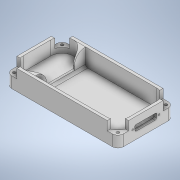
# Autodesk Inventor part: Podstawa
Saved by Autodesk Inventor 2020.3 (Build 243373000, 373)
## iProperties
Created: 2021-03-04
Part Number: Podstawa
Material: Generic
Document SubType Name: Modeling
Designer: patry
Density: 1 g/cm^3
Appearance: Default
Author: patry
Autodesk Inventor part; units mm, degrees
ref_plane "YZ Plane" through (0, 0, 0) normal (1, 0, 0) x (0, 1, 0)
ref_plane "XZ Plane" through (0, 0, 0) normal (0, 1, 0) x (-1, 0, 0)
ref_plane "XY Plane" through (0, 0, 0) normal (0, 0, 1) x (1, 0, 0)
sketch "Sketch2" plane through (0, 0, 0) normal (0, 1, 0) x (-1, 0, 0)
  line L0 (0, 0) -> (-200, 0)
  line L1 (-200, 0) -> (-200, -100)
  line L2 (-200, -100) -> (0, -100)
  line L3 (0, -100) -> (0, 0)
  dimension "d0" = 200
  dimension "d1" = 100
  constraints: 8 end point, 2 parallel, 1 horizontal, 1 perpendicular
  measures "d0" distance of L2.end L1.end
  measures "d1" distance of L1.end L0.end
extrude "Extrusion1" add sketch "Sketch2" along normal blind 11
sketch "Sketch3" plane through (0, 11, 0) normal (0, 1, 0) x (1, 0, 0)
  line L0 (0, 100) -> (0, 0) projected
  line L1 (0, 0) -> (200, 0) projected
  line L2 (0, 100) -> (200, 100)
  line L3 (200, 100) -> (200, 0)
  line L4 (200, 0) -> (0, 0)
  line L5 (0, 0) -> (0, 100)
  line L6 (0, 100) -> (5, 100)
  line L7 (5, 100) -> (5, 95)
  line L8 (5, 95) -> (0, 95)
  line L9 (0, 95) -> (0, 100)
  line L10 (200, 0) -> (195, 0)
  line L11 (195, 0) -> (195, 5)
  line L12 (195, 5) -> (200, 5)
  line L13 (200, 5) -> (200, 0)
  line L14 (5, 95) -> (195, 95)
  line L15 (195, 95) -> (195, 5)
  line L16 (195, 5) -> (5, 5)
  line L17 (5, 5) -> (5, 95)
  dimension "d4" = 5
  dimension "d5" = 5
  dimension "d6" = 5
  dimension "d7" = 5
  constraints: 32 end point, 8 parallel, 4 horizontal, 4 perpendicular
  measures "d4" distance of L7.end L8.end
  measures "d5" distance of L6.end L7.end
  measures "d6" distance of L11.end L12.end
  measures "d7" distance of L10.end L11.end
extrude "Extrusion2" add sketch "Sketch3" along normal blind 25 contours L2 L7 L8 L0 | L8 L17 L16 L11 L1 L0 | L2 L3 L12 L15 L14 L7 | L11 L12 L3 L1
fillet "Fillet1" radius 10 4 edges at (0, 18, -100) (0, 18, 0) (200, 18, 0) (200, 18, -100)
fillet "Fillet2" radius 20 4 edges at (5, 23.5, -95) (5, 23.5, -5) (195, 23.5, -5) (195, 23.5, -95)
sketch "Sketch4" plane through (0, 36, 0) normal (0, 1, 0) x (1, 0, 0)
  line L0 (0, 0) -> (200, 0)
  line L1 (200, 0) -> (200, 100)
  line L2 (200, 100) -> (0, 100)
  line L3 (0, 100) -> (0, 0)
  line L4 (0, 0) -> (7, 0)
  line L5 (7, 0) -> (7, 7)
  line L6 (7, 7) -> (0, 7)
  line L7 (0, 7) -> (0, 0)
  line L8 (200, 100) -> (193, 100)
  line L9 (193, 100) -> (193, 93)
  line L10 (193, 93) -> (200, 93)
  line L11 (200, 93) -> (200, 100)
  line L12 (7, 7) -> (193, 7)
  line L13 (193, 7) -> (193, 93)
  line L14 (193, 93) -> (7, 93)
  line L15 (7, 93) -> (7, 7)
  dimension "d12" = 200
  dimension "d13" = 100
  dimension "d14" = 7
  dimension "d15" = 7
  dimension "d16" = 7
  dimension "d17" = 7
  constraints: 32 end point, 8 parallel, 4 horizontal, 4 perpendicular
  measures "d12" distance of L2.end L1.end
  measures "d13" distance of L1.end L0.end
  measures "d14" distance of L6.end L5.end
  measures "d15" distance of L5.end L4.end
  measures "d16" distance of L10.end L9.end
  measures "d17" distance of L9.end L8.end
hole "Hole1" at (7, 36, -7) at (7, 36, -93) at (193, 36, -93) at (193, 36, -7) direction (0, -1, 0) diameter 5 end through all
sketch "Sketch6" plane through (200, 0, -10) normal (1, 0, 0) x (0, 0, -1)
  line L0 (0, 36) -> (0, 0) projected
  line L1 (80, 0) -> (0, 0) projected
  line L2 (0, 36) -> (80, 36)
  line L3 (80, 36) -> (80, 0)
  line L4 (80, 0) -> (0, 0)
  line L5 (0, 0) -> (0, 36)
  line L6 (0, 36) -> (13.5, 36)
  line L7 (13.5, 36) -> (13.5, 24.25)
  line L8 (13.5, 24.25) -> (0, 24.25)
  line L9 (0, 24.25) -> (0, 36)
  line L10 (80, 0) -> (66.5, 0)
  line L11 (66.5, 0) -> (66.5, 11.75)
  line L12 (66.5, 11.75) -> (80, 11.75)
  line L13 (80, 11.75) -> (80, 0)
  line L14 (13.5, 24.25) -> (66.5, 24.25)
  line L15 (66.5, 24.25) -> (66.5, 11.75)
  line L16 (66.5, 11.75) -> (13.5, 11.75)
  line L17 (13.5, 11.75) -> (13.5, 24.25)
  line L18 (13.5, 24.25) -> (16.5, 24.25)
  line L19 (16.5, 24.25) -> (16.5, 11.75)
  line L20 (16.5, 11.75) -> (13.5, 11.75)
  line L21 (13.5, 11.75) -> (13.5, 24.25)
  line L22 (66.5, 24.25) -> (63.5, 24.25)
  line L23 (63.5, 24.25) -> (63.5, 11.75)
  line L24 (63.5, 11.75) -> (66.5, 11.75)
  line L25 (66.5, 11.75) -> (66.5, 24.25)
  line L26 (13.5, 24.25) -> (16.5, 24.25)
  line L27 (16.5, 24.25) -> (16.5, 18)
  line L28 (16.5, 18) -> (13.5, 18)
  line L29 (13.5, 18) -> (13.5, 24.25)
  line L30 (66.5, 24.25) -> (63.5, 24.25)
  line L31 (63.5, 24.25) -> (63.5, 18)
  line L32 (63.5, 18) -> (66.5, 18)
  line L33 (66.5, 18) -> (66.5, 24.25)
  circle A0 centre (16.5, 18) radius 1.5
  circle A1 centre (63.5, 18) radius 1.5
  line L34 (13.5, 24.25) -> (19.5, 24.25)
  line L35 (19.5, 24.25) -> (19.5, 23.25)
  line L36 (19.5, 23.25) -> (13.5, 23.25)
  line L37 (13.5, 23.25) -> (13.5, 24.25)
  line L38 (66.5, 11.75) -> (60.5, 11.75)
  line L39 (60.5, 11.75) -> (60.5, 12.75)
  line L40 (60.5, 12.75) -> (66.5, 12.75)
  line L41 (66.5, 12.75) -> (66.5, 11.75)
  line L42 (60.5, 12.75) -> (19.5, 12.75)
  line L43 (19.5, 12.75) -> (19.5, 23.25)
  line L44 (19.5, 23.25) -> (60.5, 23.25)
  line L45 (60.5, 23.25) -> (60.5, 12.75)
  line L46 (19.5, 12.75) -> (21, 12.75)
  line L47 (21, 12.75) -> (21, 14.25)
  line L48 (21, 14.25) -> (19.5, 14.25)
  line L49 (19.5, 14.25) -> (19.5, 12.75)
  line L50 (60.5, 12.75) -> (59, 12.75)
  line L51 (59, 12.75) -> (59, 14.25)
  line L52 (59, 14.25) -> (60.5, 14.25)
  line L53 (60.5, 14.25) -> (60.5, 12.75)
  line L54 (19.5, 23.25) -> (21, 12.75)
  line L55 (59, 12.75) -> (60.5, 23.25)
  line L56 (16.5, 18) -> (16.5, 20.35)
  line L57 (16.5, 18) -> (17.675, 20.0352)
  line L58 (16.5, 18) -> (18.85, 18) construction
  line L59 (18.85, 19.3568) -> (18.85, 16.6432)
  line L60 (18.85, 16.6432) -> (16.5, 15.2865)
  line L61 (16.5, 15.2865) -> (14.15, 16.6432)
  line L62 (14.15, 16.6432) -> (14.15, 19.3568)
  line L63 (14.15, 19.3568) -> (16.5, 20.7135)
  line L64 (16.5, 20.7135) -> (18.85, 19.3568)
  line L65 (65.85, 19.3568) -> (65.85, 16.6432)
  line L66 (65.85, 16.6432) -> (63.5, 15.2865)
  line L67 (63.5, 15.2865) -> (61.15, 16.6432)
  line L68 (61.15, 16.6432) -> (61.15, 19.3568)
  line L69 (61.15, 19.3568) -> (63.5, 20.7135)
  line L70 (63.5, 20.7135) -> (65.85, 19.3568)
  line L71 (14.15, 19.3568) -> (14.15, 16.6432)
  line L72 (16.5, 15.2865) -> (14.15, 16.6432)
  line L73 (19.5, 12.75) -> (20.5, 12.75)
  line L74 (20.5, 12.75) -> (20.5, 13.75)
  line L75 (20.5, 13.75) -> (19.5, 13.75)
  line L76 (19.5, 13.75) -> (19.5, 12.75)
  line L77 (19.5, 13.75) -> (60.5, 13.75)
  line L78 (21, 12.75) -> (21.5, 12.75)
  line L79 (19.5, 23.25) -> (20, 23.25)
  line L80 (20, 23.25) -> (21.5, 12.75)
  line L81 (60.5, 23.25) -> (60, 23.25)
  line L82 (59, 12.75) -> (58.5, 12.75)
  line L83 (58.5, 12.75) -> (60, 23.25)
  point P0 (-10, 0)
  point P1 (59, 12.75)
  point P2 (14.15, 18)
  point P3 (20.8571, 13.75)
  point P4 (59.1429, 13.75)
  point P5 (58.6429, 13.75)
  point P6 (21.3571, 13.75)
  dimension "d123" = 186
  dimension "d124" = 86
  dimension "d31" = 36
  dimension "d32" = 80
  dimension "d33" = 13.5
  dimension "d34" = 11.75
  dimension "d35" = 13.5
  dimension "d36" = 11.75
  dimension "d37" = 3
  dimension "d38" = 3
  dimension "d39" = 3
  dimension "d40" = 6.25
  dimension "d41" = 3
  dimension "d42" = 6.25
  dimension "d43" = 3
  dimension "d44" = 3
  dimension "d45" = 6
  dimension "d46" = 1
  dimension "d47" = 6
  dimension "d48" = 1
  dimension "d49" = 1.5
  dimension "d50" = 1.5
  dimension "d51" = 1.5
  dimension "d52" = 1.5
  dimension "d141" = 2.35
  dimension "d142" = 2.35
  dimension "d143" = 60
  dimension "d144" = 1
  dimension "d145" = 1
  dimension "d148" = 0.5
  dimension "d149" = 0.5
  dimension "d150" = 0.5
  dimension "d151" = 0.5
  constraints: 164 end point, 28 parallel, 15 horizontal, 15 perpendicular, 8 point on line, 3 coincident, 2 centre point, 1 equal length, 1 midpoint, 13 other
  measures "d31" distance of L0.start L0.end
  measures "d32" distance of L0.start L2.end
  measures "d33" distance of L7.end L8.end
  measures "d34" distance of L6.end L7.end
  measures "d35" distance of L11.end L12.end
  measures "d36" distance of L10.end L11.end
  measures "d37" distance of L19.end L20.end
  measures "d38" distance of L24.end L23.end
  measures "d39" distance of L27.end L28.end
  measures "d40" distance of L26.end L27.end
  measures "d41" distance of L32.end L31.end
  measures "d42" distance of L31.end L30.end
  measures "d43" diameter of A0
  measures "d44" diameter of A1
  measures "d45" distance of L35.end L36.end
  measures "d46" distance of L34.end L35.end
  measures "d47" distance of L39.end L40.end
  measures "d48" distance of L38.end L39.end
  measures "d49" distance of L48.end L47.end
  measures "d50" distance of L47.end L46.end
  measures "d51" distance of L51.end L52.end
  measures "d52" distance of L50.end L51.end
  measures "d141" distance of L56.start L56.end
  measures "d142" distance of L56.start L57.end
  measures "d143" angle of L58 L57
  measures "d144" distance of L75.end L74.end
  measures "d145" distance of L74.end L73.end
  measures "d148" distance of L46.end L78.end
  measures "d149" distance of L35.end L79.end
  measures "d150" distance of L44.end L81.end
  measures "d151" distance of L50.end L82.end
sketch "Sketch7" plane through (0, 11, 0) normal (0, 1, 0) x (1, 0, 0)
  arc A0 (25, 95) -> (5, 75) centre (25, 75) ccw projected
  line L0 (195, 25) -> (195, 75) projected
  line L1 (5, 75) -> (195, 75)
  line L2 (195, 75) -> (195, 25)
  line L3 (195, 25) -> (5, 25)
  line L4 (5, 25) -> (5, 75)
  arc A1 (175, 5) -> (195, 25) centre (175, 25) ccw projected
  line L5 (195, 25) -> (156.55, 25)
  line L6 (156.55, 25) -> (156.55, 50)
  line L7 (156.55, 50) -> (195, 50)
  line L8 (195, 50) -> (195, 25)
  line L9 (156.55, 50) -> (149.05, 50)
  line L10 (156.55, 50) -> (152.8, 50)
  line L11 (152.8, 50) -> (152.8, 51)
  line L12 (152.8, 51) -> (156.55, 51)
  line L13 (156.55, 51) -> (156.55, 50)
  line L14 (152.8, 50) -> (21.8, 50)
  line L15 (152.8, 50) -> (283.8, 50) construction
  circle A2 centre (21.8, 50) radius 6
  line L16 (21.8, 50) -> (5.7, 50)
  line L17 (5, 32.7) -> (5, 67.3)
  circle A3 centre (25, 75) radius 20
  arc A4 (5, 25) -> (25, 5) centre (25, 25) ccw projected
  circle A5 centre (25, 25) radius 20
  line L18 (45, 108.4163) -> (45, -35.3074)
  line L19 (25, 95) -> (175, 95) projected
  line L20 (25, 95) -> (45, 95)
  line L21 (175, 5) -> (25, 5) projected
  line L22 (25, 5) -> (45, 5)
  line L23 (45, 95) -> (47, 95)
  line L24 (47, 95) -> (47, 93)
  line L25 (47, 93) -> (45, 93)
  line L26 (45, 93) -> (45, 95)
  line L27 (47, 95) -> (45, 95)
  line L28 (45, 95) -> (45, 5)
  line L29 (45, 5) -> (47, 5)
  line L30 (47, 5) -> (47, 95)
  point P0 (0, 0)
  point P1 (47, 25)
  point P2 (45, 25)
  point P3 (45, 75)
  point P4 (47, 75)
  point P5 (25, 5)
  point P6 (45, 25)
  point P7 (45, 75)
  dimension "d56" = 50
  dimension "d57" = 38.45
  dimension "d58" = 25
  dimension "d59" = 7.5
  dimension "d60" = 3.75
  dimension "d61" = 1
  dimension "d63" = 180
  dimension "d64" = 12
  dimension "d115" = 2
  dimension "d116" = 2
  constraints: 56 end point, 10 parallel, 9 horizontal, 5 perpendicular, 4 point on line, 3 centre point, 3 coincident, 1 collinear, 1 concentric, 1 tangent, 1 vertical
  measures "d56" distance of L3.end L1.start
  measures "d57" distance of L6.end L7.end
  measures "d58" distance of L5.end L6.end
  measures "d59" distance of L6.end L9.end
  measures "d60" distance of L11.end L12.end
  measures "d61" distance of L10.end L11.end
  measures "d63" angle of L14 L15
  measures "d64" diameter of A2
  measures "d115" distance of L24.end L25.end
  measures "d116" distance of L23.end L24.end
extrude "Extrusion7" add sketch "Sketch7" along normal blind 25 contours L19 L18 A3 | L18 L25 L30 L1 | L19 L24 L25 L18 | L18 L21 A5 | L3 L30 L21 L18
fillet "Fillet6" radius 20 2 edges at (46, 36, -25) (46, 36, -75)
sketch "Sketch12" plane through (0, 0, 0) normal (0, -1, 0) x (1, 0, 0)
  circle A0 centre (193, -93) radius 2.5 projected
  line L0 (193, -93) -> (193, -97)
  circle A1 centre (7, -7) radius 2.5 projected
  line L1 (193, -93) -> (7, -93)
  line L2 (7, -93) -> (7, -7)
  line L3 (7, -7) -> (193, -7)
  line L4 (193, -7) -> (193, -93)
  line L5 (193, -97) -> (7, -97)
  line L6 (7, -97) -> (7, -11)
  line L7 (7, -11) -> (193, -11)
  line L8 (193, -11) -> (193, -97)
  line L9 (190.6906, -97) -> (188.3812, -93)
  line L10 (188.3812, -93) -> (190.6906, -89)
  line L11 (190.6906, -89) -> (195.3094, -89)
  line L12 (195.3094, -89) -> (197.6188, -93)
  line L13 (197.6188, -93) -> (195.3094, -97)
  line L14 (195.3094, -97) -> (190.6906, -97)
  line L15 (190.6906, -11) -> (188.3812, -7)
  line L16 (188.3812, -7) -> (190.6906, -3)
  line L17 (190.6906, -3) -> (195.3094, -3)
  line L18 (195.3094, -3) -> (197.6188, -7)
  line L19 (197.6188, -7) -> (195.3094, -11)
  line L20 (195.3094, -11) -> (190.6906, -11)
  line L21 (4.6906, -11) -> (2.3812, -7)
  line L22 (2.3812, -7) -> (4.6906, -3)
  line L23 (4.6906, -3) -> (9.3094, -3)
  line L24 (9.3094, -3) -> (11.6188, -7)
  line L25 (11.6188, -7) -> (9.3094, -11)
  line L26 (9.3094, -11) -> (4.6906, -11)
  line L27 (4.6906, -97) -> (2.3812, -93)
  line L28 (2.3812, -93) -> (4.6906, -89)
  line L29 (4.6906, -89) -> (9.3094, -89)
  line L30 (9.3094, -89) -> (11.6188, -93)
  line L31 (11.6188, -93) -> (9.3094, -97)
  line L32 (9.3094, -97) -> (4.6906, -97)
  point P0 (0, 0)
  dimension "d122" = 4
  dimension "d123" = 186
  dimension "d124" = 86
  dimension "d125" = 186
  dimension "d126" = 86
  constraints: 66 end point, 4 coincident, 4 midpoint, 4 parallel, 2 horizontal, 2 perpendicular, 1 vertical, 52 other
  measures "d122" distance of L0.start L0.end
  measures "d123" distance of L0.start L1.end
  measures "d124" distance of L1.end L2.end
  measures "d125" distance of L6.end L7.end
  measures "d126" distance of L5.end L6.end
sketch "Sketch13" plane through (0, 36, 0) normal (0, 1, 0) x (1, 0, 0)
  arc A0 (5, 25) -> (25, 5) centre (25, 25) ccw projected
  circle A1 centre (25, 25) radius 20
  arc A2 (0, 10) -> (10, 0) centre (10, 10) ccw projected
  circle A3 centre (10, 10) radius 10
  line L0 (5.8856, 19.1144) -> (0, 19.1144)
  line L1 (0, 90) -> (0, 10) projected
  line L2 (19.1144, 5.8856) -> (19.1144, 0)
  line L3 (10, 0) -> (190, 0) projected
  line L4 (0, 19.1144) -> (19.1144, 19.1144)
  line L5 (19.1144, 19.1144) -> (19.1144, 0)
  line L6 (19.1144, 0) -> (0, 0)
  line L7 (0, 0) -> (0, 19.1144)
  arc A4 (45, 75) -> (5, 75) centre (25, 75) ccw projected
  circle A5 centre (25, 75) radius 20
  line L8 (25, 75) -> (25, 25)
  line L9 (25, 75) -> (35, 75)
  line L10 (35, 75) -> (35, 50)
  line L11 (35, 50) -> (25, 50)
  line L12 (25, 50) -> (25, 75)
  circle A6 centre (25, 75) radius 20
  circle A7 centre (10, 90) radius 10
  line L13 (0, 80.8856) -> (19.1144, 80.8856)
  line L14 (19.1144, 80.8856) -> (19.1144, 100)
  line L15 (19.1144, 100) -> (0, 100)
  line L16 (0, 100) -> (0, 80.8856)
  line L17 (0, 100) -> (200, 100)
  line L18 (200, 100) -> (200, 0)
  line L19 (200, 0) -> (0, 0)
  line L20 (0, 0) -> (0, 100)
  line L21 (0, 100) -> (100, 100)
  line L22 (100, 100) -> (100, 0)
  line L23 (100, 0) -> (0, 0)
  line L24 (0, 0) -> (0, 100)
  arc A8 (175, 5) -> (195, 25) centre (175, 25) ccw
  circle A9 centre (175, 25) radius 20
  arc A10 (190, 0) -> (200, 10) centre (190, 10) ccw
  circle A11 centre (190, 10) radius 10
  line L25 (194.1144, 19.1144) -> (200, 19.1144)
  line L26 (200, 90) -> (200, 10)
  line L27 (180.8856, 5.8856) -> (180.8856, 0)
  line L28 (200, 19.1144) -> (180.8856, 19.1144)
  line L29 (180.8856, 19.1144) -> (180.8856, 0)
  line L30 (180.8856, 0) -> (200, 0)
  line L31 (200, 0) -> (200, 19.1144)
  arc A12 (195, 75) -> (155, 75) centre (175, 75) ccw
  circle A13 centre (175, 75) radius 20
  line L32 (175, 75) -> (175, 25)
  line L33 (175, 75) -> (165, 75)
  line L34 (165, 75) -> (165, 50)
  line L35 (165, 50) -> (175, 50)
  line L36 (175, 50) -> (175, 75)
  circle A14 centre (175, 75) radius 20
  line L37 (180.8856, 80.8856) -> (180.8856, 100)
  line L38 (200, 80.8856) -> (180.8856, 80.8856)
  line L39 (200, 100) -> (200, 80.8856)
  line L40 (180.8856, 100) -> (200, 100)
  circle A15 centre (190, 90) radius 10
  line L41 (200, 0) -> (200, 100)
  line L42 (200, 0) -> (200, 100)
  point P0 (19.1144, 5.8856)
  point P1 (5.8856, 19.1144)
  point P2 (10, 100)
  point P3 (5.8856, 80.8856)
  point P4 (19.1144, 94.1144)
  point P5 (180.8856, 5.8856)
  point P6 (180.8856, 94.1144)
  point P7 (194.1144, 80.8856)
  point P8 (190, 100)
  dimension "d131" = 10
  dimension "d132" = 25
  dimension "d133" = 200
  dimension "d134" = 100
  dimension "d135" = 100
  dimension "d136" = 100
  constraints: 82 end point, 35 symmetric about line, 14 point on circle, 13 centre point, 8 parallel, 6 coincident, 5 horizontal, 5 perpendicular, 3 point on line, 1 vertical, 10 other
  measures "d131" distance of L10.end L11.end
  measures "d132" distance of L9.end L10.end
  measures "d133" distance of L18.end L19.end
  measures "d134" distance of L17.end L18.end
  measures "d135" distance of L22.end L23.end
  measures "d136" distance of L21.end L22.end
extrude "Extrusion9" cut sketch "Sketch13" against normal blind 16 contours A0 A3 A2 | A3 L1 L0 | L2 L3 A3 | L1 A7 L13 | A7 A4 | L27 A11 L3 | L15 L14 A7 | A11 A8 A10 | L17 A15 L37 | A11 L25 L18 | A15 A12 | L18 L38 A15
sketch "Sketch15" plane through (0, 11, 0) normal (0, 1, 0) x (1, 0, 0)
  line L0 (47, 95) -> (175, 95) projected
  line L1 (195, 25) -> (195, 75) projected
  line L2 (47, 95) -> (195, 95)
  line L3 (195, 95) -> (195, 52.6168)
  line L4 (195, 52.6168) -> (47, 52.6168)
  line L5 (47, 52.6168) -> (47, 95)
  line L6 (47, 5) -> (175, 5) projected
  line L7 (47, 5) -> (195, 5)
  line L8 (195, 5) -> (195, 52.6168)
  line L9 (195, 52.6168) -> (47, 52.6168)
  line L10 (47, 52.6168) -> (47, 5)
  arc A0 (175, 5) -> (195, 25) centre (175, 25) ccw projected
  circle A1 centre (175, 25) radius 20
  arc A2 (195, 75) -> (175, 95) centre (175, 75) ccw projected
  circle A3 centre (175, 75) radius 20
  point P0 (0, 0)
  constraints: 16 end point, 4 parallel, 2 centre point, 2 coincident, 2 horizontal, 2 perpendicular, 1 point on line
extrude "Extrusion10" cut sketch "Sketch15" against normal blind 6 contours L0 A3 L1 L4 L5 | A2 A3 | L4 L1 A1 L6 L10 | A0 A1
fillet "Fillet7" radius 2 1 edges at (47, 11, -50)
fillet "Fillet8" radius 4 1 edges at (47, 5, -50)
extrude "Extrusion13" cut sketch "Sketch6" against normal up to surface (5 mm away) contours L44 L80 L77 L47 L48 L54 | L44 L83 L77 L80 | L48 L47 L77 L54 | A0 L19 L28 | L28 L19 A0 | A1 L32 L23 | L23 A1 | L44 L55 L52 L51 L77 L83 | L80 L42 L47 L77 | L77 L83 L42 L80 | L77 L47 L54 | A0 L57 L19 | A0 L19 L57 | A1 L23 L32 | L42 L83 L77 L51 | L51 L77 L55 | L51 L52 L55 L77
sketch "Sketch17" plane through (195, 36, -75) normal (-1, 0, 0) x (0, 0, 1)
  circle A0 centre (1.5, -18) radius 1.5 projected
  line L0 (1.4125, -18.2016) -> (2.7875, -15.82)
  line L1 (4.1625, -16.6138) -> (4.1625, -19.7893)
  line L2 (4.1625, -19.7893) -> (1.4125, -21.377)
  line L3 (1.4125, -21.377) -> (-1.3375, -19.7893)
  line L4 (-1.3375, -19.7893) -> (-1.3375, -16.6138)
  line L5 (-1.3375, -16.6138) -> (1.4125, -15.0261)
  line L6 (1.4125, -15.0261) -> (4.1625, -16.6138)
  circle A1 centre (48.5, -18) radius 1.5 projected
  circle A2 centre (48.5, -18) radius 1.5
  line L7 (51.25, -16.6138) -> (51.25, -19.7893)
  line L8 (51.25, -19.7893) -> (48.5, -21.377)
  line L9 (48.5, -21.377) -> (45.75, -19.7893)
  line L10 (45.75, -19.7893) -> (45.75, -16.6138)
  line L11 (45.75, -16.6138) -> (48.5, -15.0261)
  line L12 (48.5, -15.0261) -> (51.25, -16.6138)
  point P0 (75, -36)
  point P1 (50, -18)
  dimension "d159" = 2.75
  constraints: 26 end point, 2 coincident, 1 centre point, 1 horizontal alignment, 1 midpoint, 13 other
  measures "d159" distance of L0.start L0.end
extrude "Extrusion14" cut sketch "Sketch17" against normal mid plane 4 contours A0 | L1 L2 L3 L4 L5 L6 | L7 L8 L9 L10 L11 L12
fillet "Fillet11" radius 2.7 4 edges at (197.5, 23.25, -29.5) (197.5, 12.75, -31) (197.5, 23.25, -70.5) (197.5, 12.75, -69)
extrude "Extrusion15" cut sketch "Sketch12" against normal blind 6 contours A0 L0 L4 | A0 L4 L11 L12 L13 L14 L0 | L4 L1 A0 | A0 L1 L10 L11 L4 | L0 L5 L9 L1 A0 | A0 L1 L0 | L7 L15 L3 L4 | L4 L3 L16 L17 L18 L19 L20
sketch "Sketch18" plane through (0, 0, 0) normal (0, -1, 0) x (1, 0, 0)
  circle A0 centre (7, -7) radius 2.5 projected
  circle A1 centre (7, -7) radius 4.25
  circle A2 centre (7, -93) radius 2.5 projected
  circle A3 centre (7, -93) radius 4.25
  point P0 (0, 0)
  dimension "d167" = 8.5
  dimension "d168" = 8.5
  constraints: 2 centre point, 2 coincident
  measures "d167" diameter of A1
  measures "d168" diameter of A3
extrude "Extrusion16" cut sketch "Sketch18" against normal blind 5 contours A0 | A1 | A2 | A3
body "Solid1"
